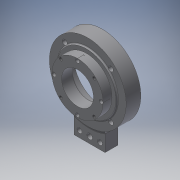
# Autodesk Inventor part: cycloid_outter_motor_side
Saved by Autodesk Inventor 2019.4 (Build 234330000, 330)
## iProperties
Created: 2019-09-11
Part Number: cycloid_outter_motor_side
Material: Generic
Document SubType Name: Modeling
Designer: cdi
Density: 1 g/cm^3
Appearance: Default
Author: cdi
Autodesk Inventor part; units mm, degrees
ref_plane "YZ Plane" through (0, 0, 0) normal (1, 0, 0) x (0, 1, 0)
ref_plane "XZ Plane" through (0, 0, 0) normal (0, 1, 0) x (-1, 0, 0)
ref_plane "XY Plane" through (0, 0, 0) normal (0, 0, 1) x (1, 0, 0)
sketch "Sketch1" plane through (0, 0, 0) normal (0, 0, 1) x (1, 0, 0)
  circle A0 centre (0, 0) radius 12.5
  circle A1 centre (0, 0) radius 19.96
  dimension "d0" = 25
  dimension "d1" = 39.92
  constraints: 2 centre point, 2 coincident
  measures "d0" diameter of A0
  measures "d1" diameter of A1
extrude "Extrusion1" add sketch "Sketch1" along normal blind 7
sketch "Sketch2" plane through (0, 0, 0) normal (0, 0, -1) x (-1, 0, 0)
  circle A0 centre (0, 0) radius 23
  circle A1 centre (0, 0) radius 12.5 projected
  dimension "d4" = 46
  constraints: 1 centre point, 1 coincident
  measures "d4" diameter of A0
extrude "Extrusion2" add sketch "Sketch2" along normal blind 2.5
sketch "Sketch3" plane through (0, 0, 7) normal (0, 0, 1) x (1, 0, 0)
  circle A0 centre (0, 18.42) radius 1.54
  line L0 (0, 0) -> (0, 23.5589)
  circle A1 centre (0, 0) radius 19.96 projected
  dimension "d7" = 3.08
  constraints: 2 end point, 1 centre point, 1 point on line, 1 tangent, 1 vertical
  measures "d7" diameter of A0
extrude "Extrusion3" cut sketch "Sketch3" against normal blind 5 contours A0 L0 | L0 A0
pattern_circular "Circular Pattern1" count 4 over 360 about axis through (0, 0, 0) along (0, 0, 1) of "Extrusion3"
sketch "Sketch4" plane through (0, 0, 0) normal (0, 0, 1) x (1, 0, 0)
  circle A0 centre (13.0249, 13.0249) radius 1.54 projected
  circle A1 centre (13.0249, -13.0249) radius 1.54 projected
  point P0 (0, 0)
  point P1 (14.1139, 14.1139)
  point P2 (-13.0249, 13.0249)
  point P3 (-13.0249, -13.0249)
  point P4 (14.1139, -14.1139)
  constraints: 2 other
hole "Hole1" [suppressed]
sketch "Sketch6" plane through (0, 0, -2.5) normal (0, 0, -1) x (-1, 0, 0)
  circle A0 centre (0, 0) radius 23 projected
  arc A1 (-12.5, 0) -> (-12.5, 0) centre (0, 0) ccw projected
  circle A2 centre (0, 0) radius 30
  dimension "d28" = 60
  constraints: 1 centre point, 1 coincident
  measures "d28" diameter of A2
extrude "Extrusion4" add sketch "Sketch6" against normal blind 1.5 contours A2
fillet "Fillet1" radius 1 1 edges at (12.5, 0, -2.5)
sketch "Sketch7" plane through (0, 0, -2.5) normal (0, 0, -1) x (-1, 0, 0)
  circle A0 centre (0, 0) radius 22.5
  circle A1 centre (0, 0) radius 30 projected
  dimension "d32" = 45
  constraints: 1 centre point, 1 coincident
  measures "d32" diameter of A0
extrude "Extrusion5" add sketch "Sketch7" along normal blind 10
sketch "Sketch8" plane through (0, 0, -12.5) normal (0, 0, -1) x (-1, 0, 0)
  circle A0 centre (0, 0) radius 30 projected
  line L0 (0, 30) -> (0, 0)
  circle A1 centre (0, 25.5) radius 1.5
  circle A2 centre (-18.0312, 18.0312) radius 1.5
  circle A3 centre (-25.5, 0) radius 1.5
  circle A4 centre (-18.0312, -18.0312) radius 1.5
  circle A5 centre (0, -25.5) radius 1.5
  circle A6 centre (18.0312, -18.0312) radius 1.5
  circle A7 centre (25.5, 0) radius 1.5
  circle A8 centre (18.0312, 18.0312) radius 1.5
  dimension "d35" = 3
  dimension "d36" = 25.5
  dimension "d39" = 360
  constraints: 8 centre point, 2 end point, 1 point on line, 1 vertical, 1 vertical alignment, 18 other
  measures "d35" diameter of A1
  measures "d36" distance of point (0, 0) A1.centre
hole "Hole3" at (-18.0312, 18.0312, -12.5) at (-18.0312, -18.0312, -12.5) at (18.0312, -18.0312, -12.5) at (18.0312, 18.0312, -12.5) direction (0, 0, 1) diameter 3.88 depth 20 tip angle 118 countersink diameter 4.34 countersink angle 7
fillet "Fillet2" radius 1 1 edges at (22.5, 0, -2.5)
sketch "Sketch9" plane through (0, 0, -12.5) normal (0, 0, -1) x (-1, 0, 0)
  line L0 (-12, -42.5) -> (-12, -22.5)
  line L1 (-12, -22.5) -> (12, -22.5)
  line L2 (12, -22.5) -> (12, -42.5)
  line L3 (12, -42.5) -> (-12, -42.5)
  line L4 (-12, -42.5) -> (12, -22.5) construction
  line L5 (-12, -22.5) -> (12, -42.5) construction
  circle A0 centre (0, 0) radius 22.5 projected
  point P0 (0, -32.5)
  dimension "d50" = 24
  dimension "d51" = 0
  dimension "d52" = 20
  constraints: 12 end point, 2 midpoint, 2 parallel, 1 perpendicular, 1 tangent, 1 vertical
  measures "d50" distance of L2.end L0.start
  measures "d51" horizontal distance of point (0, 0) point (0, -32.5)
  measures "d52" distance of L1.end L2.end
extrude "Extrusion6" add sketch "Sketch9" against normal blind 10 contours L0 L1 L2 L3
fillet "Fillet3" radius 4 2 edges at (12, -27.4955, -7.5) (-12, -27.4955, -7.5)
sketch "Sketch10" plane through (0, 0, -2.5) normal (0, 0, 1) x (1, 0, 0)
  circle A0 centre (0, -37.5) radius 1.5
  line L0 (-12, -42.5) -> (12, -42.5) projected
  point P0 (0, 0)
  dimension "d56" = 3
  dimension "d57" = 5
  constraints: 1 centre point
  measures "d56" diameter of A0
  measures "d57" distance from line of L0 A0.centre
hole "Hole4" at (0, -37.5, -2.5) direction (0, 0, -1) diameter 3.88 depth 10 tip angle 118 countersink diameter 4.34 countersink angle 7
sketch "Sketch11" plane through (0, 0, -12.5) normal (0, 0, -1) x (-1, 0, 0)
  circle A0 centre (8, -37.5) radius 1.5
  line L0 (12, -42.5) -> (-12, -42.5) projected
  circle A1 centre (0, -37.5) radius 1.94 projected
  point P0 (0, 0)
  dimension "d65" = 3
  dimension "d66" = 5
  dimension "d67" = 8
  constraints: 1 centre point
  measures "d65" diameter of A0
  measures "d66" distance from line of L0 A0.centre
  measures "d67" distance of A1.centre A0.centre
hole "Hole5" at (-8, -37.5, -12.5) direction (0, 0, 1) diameter 3.88 depth 10 tip angle 118 countersink diameter 4.34 countersink angle 7
mirror "Mirror1" about plane through (0, 0, 0) normal (1, 0, 0) of "Hole5"
fillet "Fillet4" radius 2.5 1 edges at (0, -30, -2.5)
fillet "Fillet5" radius 1 1 edges at (23, 0, -1)
sketch "Sketch12" plane through (0, 18.42, 7) normal (0, 0, 1) x (1, 0, 0)
  circle A0 centre (0, 0) radius 1.54 projected
  circle A1 centre (0, -18.42) radius 18.42
  line L0 (0, -18.42) -> (0, 0)
  line L1 (0, -18.42) -> (-21.1028, 2.6828)
  circle A2 centre (-13.0249, -5.3951) radius 1.5
  point P0 (0, 1.54)
  dimension "d77" = 45
  dimension "d78" = 3
  constraints: 4 end point, 2 centre point, 2 point on circle, 1 coincident, 1 point on line, 1 vertical, 1 vertical alignment
  measures "d77" angle of L0 L1
  measures "d78" diameter of A2
hole "Hole6" at (-13.0249, 13.0249, 7) direction (0, 0, -1) diameter 2.459 end through all thread size "M3x0.5" class "6H" standard "ISO Metric profile"
pattern_circular "Circular Pattern2" count 4 over 360 about axis through (0, 0, 0) along (0, 0, 1) of "Hole6"
body "Solid1"
